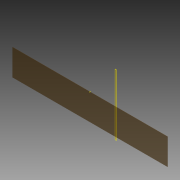
# Autodesk Inventor part: FE-PlayerStationBottom
Saved by Autodesk Inventor 2013 (Build 170138000, 138)
## iProperties
Created: 2013-01-14
Part Number: FE-PlayerStationBottom
Material: Polycarbonate, Smoke
Document SubType Name: Modeling
Designer: Phillip
Density: 1 g/cm^3
Author: Phillip
Autodesk Inventor part; units mm, degrees
ref_plane "YZ Plane" through (0, 0, 0) normal (1, 0, 0) x (0, 1, 0)
ref_plane "XZ Plane" through (0, 0, 0) normal (0, 1, 0) x (-1, 0, 0)
ref_plane "XY Plane" through (0, 0, 0) normal (0, 0, 1) x (1, 0, 0)
ref_plane "Work Plane1" through (1828.8, 0, 0) normal (0, 0, 1) x (1, 0, 0)
sketch "Sketch1" plane through (1828.8, 0, 0) normal (0, 0, 1) x (1, 0, 0)
  line L0 (-6607.9116, 2.5527) -> (4823.5616, 2.5527)
  line L1 (-1812.925, 1986.1022) -> (-3654.425, 1986.1022) projected
  line L2 (-3648.1338, 933.4627) -> (1870.075, 933.4627)
  line L3 (1870.075, 933.4627) -> (1870.075, 0)
  line L4 (1870.075, 0) -> (-3648.1338, 0)
  line L5 (-3648.1338, 0) -> (-3648.1338, 933.4627)
  line L6 (1870.075, 1986.1022) -> (1870.075, 3052.9022) projected
  line L7 (1870.075, 1986.1022) -> (1870.075, 3052.9022) projected
  line L8 (1870.075, 3052.9022) -> (28.575, 3052.9022) projected
  line L9 (44.45, 0) -> (0, 0) projected
  line L10 (44.45, 0) -> (44.45, 1981.2) projected
  line L11 (0, 1981.2) -> (44.45, 1981.2) projected
  line L12 (0, 0) -> (0, 1981.2) projected
  line L13 (18.9865, 1998.8657) -> (-1803.3365, 1998.8657) projected
  line L14 (1870.075, 1981.2) -> (-3654.425, 1981.2) projected
  line L15 (1870.075, 1981.2) -> (-3654.425, 1981.2) projected
  line L16 (-3615.69, 933.4627) -> (-1828.8, 933.4627) projected
  point P0 (-1828.8, 0)
  constraints: 10 end point, 3 collinear, 1 horizontal, 1 parallel, 1 perpendicular, 2 other
extrude "Extrusion1" add sketch "Sketch1" along normal blind 6.35 contours L5 L2 L12 L0 | L0 L12 L4 L5 | L12 L2 L10 L0 | L0 L10 L4 L12 | L10 L2 L3 L0 | L0 L3 L4 L10
ref_plane "Work Plane2" through (939.7706, 933.4627, 6.35) normal (-1, 0, 0) x (0, -1, 0)
body "Solid1"
